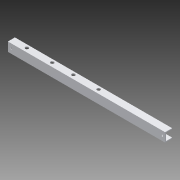
# Autodesk Inventor part: Shooter Frame - CIM Mount
Saved by Autodesk Inventor 2013 (Build 170138000, 138)
## iProperties
Created: 2013-01-08
Part Number: Shooter Frame - CIM Mount
Material: Aluminum 6061
Document SubType Name: Modeling
Designer: Naphat
Density: 2.71 g/cm^3
Mass: 341.078 g
Surface Area: 882.87 cm^2
Volume: 125.859 cm^3
Author: Naphat
Autodesk Inventor part; units mm, degrees
ref_plane "YZ Plane" through (0, 0, 0) normal (1, 0, 0) x (0, 1, 0)
ref_plane "XZ Plane" through (0, 0, 0) normal (0, 1, 0) x (-1, 0, 0)
ref_plane "XY Plane" through (0, 0, 0) normal (0, 0, 1) x (1, 0, 0)
sketch "Sketch1" plane through (0, 0, 0) normal (0, 0, 1) x (1, 0, 0)
  line L0 (-16, 12.5) -> (-13, 12.5)
  line L1 (-13, 12.5) -> (-13, -9.5)
  line L2 (-13, -9.5) -> (13, -9.5)
  line L3 (13, -9.5) -> (13, 12.5)
  line L4 (13, 12.5) -> (16, 12.5)
  line L5 (16, 12.5) -> (16, -12.5)
  line L6 (16, -12.5) -> (-16, -12.5)
  line L7 (-16, -12.5) -> (-16, 12.5)
  point P0 (0, 0)
  dimension "d0" = 3
  dimension "d2" = 3
  dimension "d3" = 25
  dimension "d4" = 32
  dimension "d5" = 16
  dimension "d7" = 12.5
  dimension "d8" = 3
  dimension "d74" = 25
  constraints: 16 end point, 5 parallel, 1 collinear, 1 horizontal, 1 perpendicular
  measures "d0" distance of L0.start L0.end
  measures "d2" distance of L3.end L4.end
  measures "d3" distance of L6.end L0.start
  measures "d4" distance of L5.end L6.end
  measures "d5" distance from line of point (0, 0) L7
  measures "d7" distance from line of L6 point (0, 0)
  measures "d8" distance between parallel lines of L6 L2
  measures "d74" distance between parallel lines of L6 L4
extrude "Extrusion1" add sketch "Sketch1" against normal blind 558.8
sketch "Sketch8" plane through (-16, -12.5, 0) normal (0, -1, 0) x (1, 0, 0)
  line L0 (32, -558.8) -> (0, -558.8) projected
  line L1 (32, 0) -> (32, -558.8) projected
  circle A0 centre (16, -547.8) radius 3.175
  line L2 (32, 0) -> (0, 0) projected
  circle A1 centre (16, -11) radius 3.175
  point P0 (16, 0)
  dimension "d114" = 6.35
  dimension "d116" = 16
  dimension "d117" = 11
  dimension "d125" = 6.35
  dimension "d126" = 11
  constraints: 2 centre point
  measures "d114" diameter of A0
  measures "d116" distance from line of A0.centre L1
  measures "d117" distance from line of A0.centre L0
  measures "d125" diameter of A1
  measures "d126" distance from line of A1.centre L2
hole "Hole5" at (0, -12.5, -547.8) at (0, -12.5, -11) direction (0, 1, 0) diameter 6.35 end through all
sketch "Sketch9" plane through (-13, -9.5, 0) normal (1, 0, 0) x (0, 0, -1)
  circle A0 centre (505.2, 11) radius 6 projected
  circle A1 centre (415.2, 11) radius 6 projected
  circle A2 centre (340.1, 11) radius 6 projected
  circle A3 centre (250.1, 11) radius 6 projected
  point P0 (0, 9.5)
hole "Hole6" at (-13, 1.5, -340.1) at (-13, 1.5, -250.1) at (-13, 1.5, -505.2) at (-13, 1.5, -415.2) direction (-1, 0, 0) diameter 12 depth 3 tip angle 118
equation "\"d2\" = d0"
equation "\"d5\" = 0.5 * d4"
equation "\"d7\" = 0.5 * d3"
equation "\"d8\" = d0"
equation "\"d74\" = d3"
equation "\"d126\" = d117"
body "Solid1"
